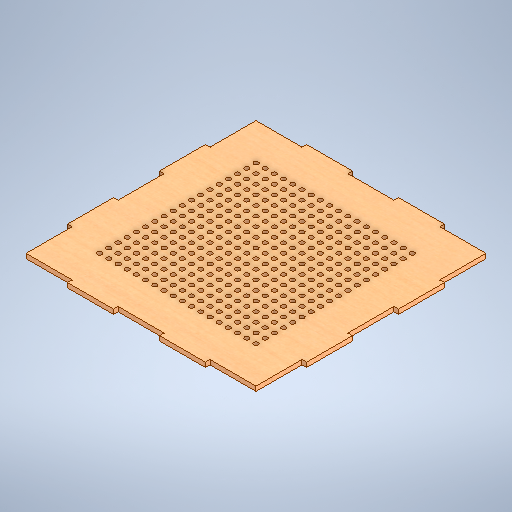
# Autodesk Inventor part: Tapa1
Saved by Autodesk Inventor 2025 (Build 290162000, 162)
## iProperties
Created: 2024-11-02
Part Number: Tapa1
Material: Wood (Cherry)
Document SubType Name: Sheet Metal
Designer: g.marin
Density: 0.63 g/cm^3
Sheet Metal Rule: Default
Appearance: Cherry - Natural Low Gloss
Author: g.marin
Autodesk Inventor part; units mm, degrees
ref_plane "YZ Plane" through (0, 0, 0) normal (1, 0, 0) x (0, 1, 0)
ref_plane "XZ Plane" through (0, 0, 0) normal (0, 1, 0) x (-1, 0, 0)
ref_plane "XY Plane" through (0, 0, 0) normal (0, 0, 1) x (1, 0, 0)
sketch "Sketch1" plane through (0, 0, 0) normal (0, 1, 0) x (-1, 0, 0)
  line L0 (-125, 125) -> (125, 125)
  line L1 (125, 125) -> (125, -125)
  line L2 (125, -125) -> (-125, -125)
  line L3 (-125, -125) -> (-125, 125)
  line L4 (-125, 125) -> (125, -125) construction
  line L5 (125, 125) -> (-125, -125) construction
  line L6 (0, 125) -> (0, -125) construction
  line L7 (125, 0) -> (-125, 0) construction
  line L8 (125, 75) -> (130, 75)
  line L9 (130, 75) -> (130, 25)
  line L10 (130, 25) -> (125, 25)
  line L11 (125, 25) -> (125, 75)
  line L12 (75, 125) -> (25, 125)
  line L13 (25, 125) -> (25, 130)
  line L14 (25, 130) -> (75, 130)
  line L15 (75, 130) -> (75, 125)
  line L16 (125, -75) -> (130, -75)
  line L17 (130, -75) -> (130, -25)
  line L18 (130, -25) -> (125, -25)
  line L19 (-125, 75) -> (-130, 75)
  line L20 (-130, 75) -> (-130, 25)
  line L21 (-130, 25) -> (-125, 25)
  line L22 (-130, -75) -> (-130, -25)
  line L23 (-125, -75) -> (-130, -75)
  line L24 (-130, -25) -> (-125, -25)
  line L25 (-25, 125) -> (-25, 130)
  line L26 (-25, 130) -> (-75, 130)
  line L27 (-75, 130) -> (-75, 125)
  line L28 (25, -125) -> (25, -130)
  line L29 (25, -130) -> (75, -130)
  line L30 (75, -130) -> (75, -125)
  line L31 (-75, -130) -> (-75, -125)
  line L32 (-25, -130) -> (-75, -130)
  line L33 (-25, -125) -> (-25, -130)
  line L34 (95, 95) -> (-95, 95)
  line L35 (-95, 95) -> (-95, -95)
  line L36 (-95, -95) -> (95, -95)
  line L37 (95, -95) -> (95, 95)
  line L38 (95, 95) -> (-95, -95) construction
  line L39 (-95, 95) -> (95, -95) construction
  circle A0 centre (85, -85) radius 2.5
  circle A1 centre (75, -85) radius 2.5
  circle A2 centre (65, -85) radius 2.5
  circle A3 centre (55, -85) radius 2.5
  circle A4 centre (45, -85) radius 2.5
  circle A5 centre (35, -85) radius 2.5
  circle A6 centre (25, -85) radius 2.5
  circle A7 centre (15, -85) radius 2.5
  circle A8 centre (5, -85) radius 2.5
  circle A9 centre (-5, -85) radius 2.5
  circle A10 centre (-15, -85) radius 2.5
  circle A11 centre (-25, -85) radius 2.5
  circle A12 centre (-35, -85) radius 2.5
  circle A13 centre (-45, -85) radius 2.5
  circle A14 centre (-55, -85) radius 2.5
  circle A15 centre (-65, -85) radius 2.5
  circle A16 centre (-75, -85) radius 2.5
  circle A17 centre (-85, -85) radius 2.5
  circle A18 centre (85, -75) radius 2.5
  circle A19 centre (75, -75) radius 2.5
  circle A20 centre (65, -75) radius 2.5
  circle A21 centre (55, -75) radius 2.5
  circle A22 centre (45, -75) radius 2.5
  circle A23 centre (35, -75) radius 2.5
  circle A24 centre (25, -75) radius 2.5
  circle A25 centre (15, -75) radius 2.5
  circle A26 centre (5, -75) radius 2.5
  circle A27 centre (-5, -75) radius 2.5
  circle A28 centre (-15, -75) radius 2.5
  circle A29 centre (-25, -75) radius 2.5
  circle A30 centre (-35, -75) radius 2.5
  circle A31 centre (-45, -75) radius 2.5
  circle A32 centre (-55, -75) radius 2.5
  circle A33 centre (-65, -75) radius 2.5
  circle A34 centre (-75, -75) radius 2.5
  circle A35 centre (-85, -75) radius 2.5
  circle A36 centre (85, -65) radius 2.5
  circle A37 centre (75, -65) radius 2.5
  circle A38 centre (65, -65) radius 2.5
  circle A39 centre (55, -65) radius 2.5
  circle A40 centre (45, -65) radius 2.5
  circle A41 centre (35, -65) radius 2.5
  circle A42 centre (25, -65) radius 2.5
  circle A43 centre (15, -65) radius 2.5
  circle A44 centre (5, -65) radius 2.5
  circle A45 centre (-5, -65) radius 2.5
  circle A46 centre (-15, -65) radius 2.5
  circle A47 centre (-25, -65) radius 2.5
  circle A48 centre (-35, -65) radius 2.5
  circle A49 centre (-45, -65) radius 2.5
  circle A50 centre (-55, -65) radius 2.5
  circle A51 centre (-65, -65) radius 2.5
  circle A52 centre (-75, -65) radius 2.5
  circle A53 centre (-85, -65) radius 2.5
  circle A54 centre (85, -55) radius 2.5
  circle A55 centre (75, -55) radius 2.5
  circle A56 centre (65, -55) radius 2.5
  circle A57 centre (55, -55) radius 2.5
  circle A58 centre (45, -55) radius 2.5
  circle A59 centre (35, -55) radius 2.5
  circle A60 centre (25, -55) radius 2.5
  circle A61 centre (15, -55) radius 2.5
  circle A62 centre (5, -55) radius 2.5
  circle A63 centre (-5, -55) radius 2.5
  circle A64 centre (-15, -55) radius 2.5
  circle A65 centre (-25, -55) radius 2.5
  circle A66 centre (-35, -55) radius 2.5
  circle A67 centre (-45, -55) radius 2.5
  circle A68 centre (-55, -55) radius 2.5
  circle A69 centre (-65, -55) radius 2.5
  circle A70 centre (-75, -55) radius 2.5
  circle A71 centre (-85, -55) radius 2.5
  circle A72 centre (85, -45) radius 2.5
  circle A73 centre (75, -45) radius 2.5
  circle A74 centre (65, -45) radius 2.5
  circle A75 centre (55, -45) radius 2.5
  circle A76 centre (45, -45) radius 2.5
  circle A77 centre (35, -45) radius 2.5
  circle A78 centre (25, -45) radius 2.5
  circle A79 centre (15, -45) radius 2.5
  circle A80 centre (5, -45) radius 2.5
  circle A81 centre (-5, -45) radius 2.5
  circle A82 centre (-15, -45) radius 2.5
  circle A83 centre (-25, -45) radius 2.5
  circle A84 centre (-35, -45) radius 2.5
  circle A85 centre (-45, -45) radius 2.5
  circle A86 centre (-55, -45) radius 2.5
  circle A87 centre (-65, -45) radius 2.5
  circle A88 centre (-75, -45) radius 2.5
  circle A89 centre (-85, -45) radius 2.5
  circle A90 centre (85, -35) radius 2.5
  circle A91 centre (75, -35) radius 2.5
  circle A92 centre (65, -35) radius 2.5
  circle A93 centre (55, -35) radius 2.5
  circle A94 centre (45, -35) radius 2.5
  circle A95 centre (35, -35) radius 2.5
  circle A96 centre (25, -35) radius 2.5
  circle A97 centre (15, -35) radius 2.5
  circle A98 centre (5, -35) radius 2.5
  circle A99 centre (-5, -35) radius 2.5
  circle A100 centre (-15, -35) radius 2.5
  circle A101 centre (-25, -35) radius 2.5
  circle A102 centre (-35, -35) radius 2.5
  circle A103 centre (-45, -35) radius 2.5
  circle A104 centre (-55, -35) radius 2.5
  circle A105 centre (-65, -35) radius 2.5
  circle A106 centre (-75, -35) radius 2.5
  circle A107 centre (-85, -35) radius 2.5
  circle A108 centre (85, -25) radius 2.5
  circle A109 centre (75, -25) radius 2.5
  circle A110 centre (65, -25) radius 2.5
  circle A111 centre (55, -25) radius 2.5
  circle A112 centre (45, -25) radius 2.5
  circle A113 centre (35, -25) radius 2.5
  circle A114 centre (25, -25) radius 2.5
  circle A115 centre (15, -25) radius 2.5
  circle A116 centre (5, -25) radius 2.5
  circle A117 centre (-5, -25) radius 2.5
  circle A118 centre (-15, -25) radius 2.5
  circle A119 centre (-25, -25) radius 2.5
  circle A120 centre (-35, -25) radius 2.5
  circle A121 centre (-45, -25) radius 2.5
  circle A122 centre (-55, -25) radius 2.5
  circle A123 centre (-65, -25) radius 2.5
  circle A124 centre (-75, -25) radius 2.5
  circle A125 centre (-85, -25) radius 2.5
  circle A126 centre (85, -15) radius 2.5
  circle A127 centre (75, -15) radius 2.5
  circle A128 centre (65, -15) radius 2.5
  circle A129 centre (55, -15) radius 2.5
  circle A130 centre (45, -15) radius 2.5
  circle A131 centre (35, -15) radius 2.5
  circle A132 centre (25, -15) radius 2.5
  circle A133 centre (15, -15) radius 2.5
  circle A134 centre (5, -15) radius 2.5
  circle A135 centre (-5, -15) radius 2.5
  circle A136 centre (-15, -15) radius 2.5
  circle A137 centre (-25, -15) radius 2.5
  circle A138 centre (-35, -15) radius 2.5
  circle A139 centre (-45, -15) radius 2.5
  circle A140 centre (-55, -15) radius 2.5
  circle A141 centre (-65, -15) radius 2.5
  circle A142 centre (-75, -15) radius 2.5
  circle A143 centre (-85, -15) radius 2.5
  circle A144 centre (85, -5) radius 2.5
  circle A145 centre (75, -5) radius 2.5
  circle A146 centre (65, -5) radius 2.5
  circle A147 centre (55, -5) radius 2.5
  circle A148 centre (45, -5) radius 2.5
  circle A149 centre (35, -5) radius 2.5
  circle A150 centre (25, -5) radius 2.5
  circle A151 centre (15, -5) radius 2.5
  circle A152 centre (5, -5) radius 2.5
  circle A153 centre (-5, -5) radius 2.5
  circle A154 centre (-15, -5) radius 2.5
  circle A155 centre (-25, -5) radius 2.5
  circle A156 centre (-35, -5) radius 2.5
  circle A157 centre (-45, -5) radius 2.5
  circle A158 centre (-55, -5) radius 2.5
  circle A159 centre (-65, -5) radius 2.5
  circle A160 centre (-75, -5) radius 2.5
  circle A161 centre (-85, -5) radius 2.5
  circle A162 centre (85, 5) radius 2.5
  circle A163 centre (75, 5) radius 2.5
  circle A164 centre (65, 5) radius 2.5
  circle A165 centre (55, 5) radius 2.5
  circle A166 centre (45, 5) radius 2.5
  circle A167 centre (35, 5) radius 2.5
  circle A168 centre (25, 5) radius 2.5
  circle A169 centre (15, 5) radius 2.5
  circle A170 centre (5, 5) radius 2.5
  circle A171 centre (-5, 5) radius 2.5
  circle A172 centre (-15, 5) radius 2.5
  circle A173 centre (-25, 5) radius 2.5
  circle A174 centre (-35, 5) radius 2.5
  circle A175 centre (-45, 5) radius 2.5
  circle A176 centre (-55, 5) radius 2.5
  circle A177 centre (-65, 5) radius 2.5
  circle A178 centre (-75, 5) radius 2.5
  circle A179 centre (-85, 5) radius 2.5
  circle A180 centre (85, 15) radius 2.5
  circle A181 centre (75, 15) radius 2.5
  circle A182 centre (65, 15) radius 2.5
  circle A183 centre (55, 15) radius 2.5
  circle A184 centre (45, 15) radius 2.5
  circle A185 centre (35, 15) radius 2.5
  circle A186 centre (25, 15) radius 2.5
  circle A187 centre (15, 15) radius 2.5
  circle A188 centre (5, 15) radius 2.5
  circle A189 centre (-5, 15) radius 2.5
  circle A190 centre (-15, 15) radius 2.5
  circle A191 centre (-25, 15) radius 2.5
  circle A192 centre (-35, 15) radius 2.5
  circle A193 centre (-45, 15) radius 2.5
  circle A194 centre (-55, 15) radius 2.5
  circle A195 centre (-65, 15) radius 2.5
  circle A196 centre (-75, 15) radius 2.5
  circle A197 centre (-85, 15) radius 2.5
  circle A198 centre (85, 25) radius 2.5
  circle A199 centre (75, 25) radius 2.5
  circle A200 centre (65, 25) radius 2.5
  circle A201 centre (55, 25) radius 2.5
  circle A202 centre (45, 25) radius 2.5
  circle A203 centre (35, 25) radius 2.5
  circle A204 centre (25, 25) radius 2.5
  circle A205 centre (15, 25) radius 2.5
  circle A206 centre (5, 25) radius 2.5
  circle A207 centre (-5, 25) radius 2.5
  circle A208 centre (-15, 25) radius 2.5
  circle A209 centre (-25, 25) radius 2.5
  circle A210 centre (-35, 25) radius 2.5
  circle A211 centre (-45, 25) radius 2.5
  circle A212 centre (-55, 25) radius 2.5
  circle A213 centre (-65, 25) radius 2.5
  circle A214 centre (-75, 25) radius 2.5
  circle A215 centre (-85, 25) radius 2.5
  circle A216 centre (85, 35) radius 2.5
  circle A217 centre (75, 35) radius 2.5
  circle A218 centre (65, 35) radius 2.5
  circle A219 centre (55, 35) radius 2.5
  circle A220 centre (45, 35) radius 2.5
  circle A221 centre (35, 35) radius 2.5
  circle A222 centre (25, 35) radius 2.5
  circle A223 centre (15, 35) radius 2.5
  circle A224 centre (5, 35) radius 2.5
  circle A225 centre (-5, 35) radius 2.5
  circle A226 centre (-15, 35) radius 2.5
  circle A227 centre (-25, 35) radius 2.5
  circle A228 centre (-35, 35) radius 2.5
  circle A229 centre (-45, 35) radius 2.5
  circle A230 centre (-55, 35) radius 2.5
  circle A231 centre (-65, 35) radius 2.5
  circle A232 centre (-75, 35) radius 2.5
  circle A233 centre (-85, 35) radius 2.5
  circle A234 centre (85, 45) radius 2.5
  circle A235 centre (75, 45) radius 2.5
  circle A236 centre (65, 45) radius 2.5
  circle A237 centre (55, 45) radius 2.5
  circle A238 centre (45, 45) radius 2.5
  circle A239 centre (35, 45) radius 2.5
  circle A240 centre (25, 45) radius 2.5
  circle A241 centre (15, 45) radius 2.5
  circle A242 centre (5, 45) radius 2.5
  circle A243 centre (-5, 45) radius 2.5
  circle A244 centre (-15, 45) radius 2.5
  circle A245 centre (-25, 45) radius 2.5
  circle A246 centre (-35, 45) radius 2.5
  circle A247 centre (-45, 45) radius 2.5
  circle A248 centre (-55, 45) radius 2.5
  circle A249 centre (-65, 45) radius 2.5
  circle A250 centre (-75, 45) radius 2.5
  circle A251 centre (-85, 45) radius 2.5
  circle A252 centre (85, 55) radius 2.5
  circle A253 centre (75, 55) radius 2.5
  circle A254 centre (65, 55) radius 2.5
  circle A255 centre (55, 55) radius 2.5
  circle A256 centre (45, 55) radius 2.5
  circle A257 centre (35, 55) radius 2.5
  circle A258 centre (25, 55) radius 2.5
  circle A259 centre (15, 55) radius 2.5
  circle A260 centre (5, 55) radius 2.5
  circle A261 centre (-5, 55) radius 2.5
  circle A262 centre (-15, 55) radius 2.5
  circle A263 centre (-25, 55) radius 2.5
  circle A264 centre (-35, 55) radius 2.5
  circle A265 centre (-45, 55) radius 2.5
  circle A266 centre (-55, 55) radius 2.5
  circle A267 centre (-65, 55) radius 2.5
  circle A268 centre (-75, 55) radius 2.5
  circle A269 centre (-85, 55) radius 2.5
  circle A270 centre (85, 65) radius 2.5
  circle A271 centre (75, 65) radius 2.5
  circle A272 centre (65, 65) radius 2.5
  circle A273 centre (55, 65) radius 2.5
  circle A274 centre (45, 65) radius 2.5
  circle A275 centre (35, 65) radius 2.5
  circle A276 centre (25, 65) radius 2.5
  circle A277 centre (15, 65) radius 2.5
  circle A278 centre (5, 65) radius 2.5
  circle A279 centre (-5, 65) radius 2.5
  circle A280 centre (-15, 65) radius 2.5
  circle A281 centre (-25, 65) radius 2.5
  circle A282 centre (-35, 65) radius 2.5
  circle A283 centre (-45, 65) radius 2.5
  circle A284 centre (-55, 65) radius 2.5
  circle A285 centre (-65, 65) radius 2.5
  circle A286 centre (-75, 65) radius 2.5
  circle A287 centre (-85, 65) radius 2.5
  circle A288 centre (85, 75) radius 2.5
  circle A289 centre (75, 75) radius 2.5
  circle A290 centre (65, 75) radius 2.5
  circle A291 centre (55, 75) radius 2.5
  circle A292 centre (45, 75) radius 2.5
  circle A293 centre (35, 75) radius 2.5
  circle A294 centre (25, 75) radius 2.5
  circle A295 centre (15, 75) radius 2.5
  circle A296 centre (5, 75) radius 2.5
  circle A297 centre (-5, 75) radius 2.5
  circle A298 centre (-15, 75) radius 2.5
  circle A299 centre (-25, 75) radius 2.5
  circle A300 centre (-35, 75) radius 2.5
  circle A301 centre (-45, 75) radius 2.5
  circle A302 centre (-55, 75) radius 2.5
  circle A303 centre (-65, 75) radius 2.5
  circle A304 centre (-75, 75) radius 2.5
  circle A305 centre (-85, 75) radius 2.5
  circle A306 centre (85, 85) radius 2.5
  circle A307 centre (75, 85) radius 2.5
  circle A308 centre (65, 85) radius 2.5
  circle A309 centre (55, 85) radius 2.5
  circle A310 centre (45, 85) radius 2.5
  circle A311 centre (35, 85) radius 2.5
  circle A312 centre (25, 85) radius 2.5
  circle A313 centre (15, 85) radius 2.5
  circle A314 centre (5, 85) radius 2.5
  circle A315 centre (-5, 85) radius 2.5
  circle A316 centre (-15, 85) radius 2.5
  circle A317 centre (-25, 85) radius 2.5
  circle A318 centre (-35, 85) radius 2.5
  circle A319 centre (-45, 85) radius 2.5
  circle A320 centre (-55, 85) radius 2.5
  circle A321 centre (-65, 85) radius 2.5
  circle A322 centre (-75, 85) radius 2.5
  circle A323 centre (-85, 85) radius 2.5
  point P0 (0, 0)
  point P1 (-25, 125)
  point P2 (-75, 125)
  point P3 (-125, -25)
  point P4 (-125, -75)
  point P5 (-75, -125)
  point P6 (-25, -125)
  point P7 (25, -125)
  point P8 (75, -125)
  point P9 (125, -75)
  point P10 (125, -25)
  point P11 (125, 25)
  dimension "d0" = 250
  dimension "d1" = 250
  dimension "d3" = 50
  dimension "d5" = 50
  dimension "d6" = 50
  dimension "d7" = 50
  dimension "d10" = 5
  dimension "d11" = 5
  dimension "d13" = 30
  dimension "d14" = 5
  dimension "d15" = 10
  dimension "d18" = 10
  dimension "d21" = 10
  constraints: 324 centre point, 80 end point, 24 symmetric about line, 8 midpoint, 8 parallel, 5 horizontal, 4 perpendicular, 4 point on line, 1 vertical, 646 other
  measures "d0" distance of L1.end L2.end
  measures "d1" distance of L0.end L1.end
  measures "d3" distance of L8.end L9.end
  measures "d5" distance between parallel lines of L15 L1
  measures "d6" distance between parallel lines of L0 L8
  measures "d7" distance of L13.end L14.end
  measures "d10" distance of L9.end L10.end
  measures "d11" distance of L12.end L13.end
  measures "d13" distance between parallel lines of L3 L35
  measures "d14" diameter of A0
  measures "d15" distance from line of A0.centre L36
  measures "d18" distance of A0.centre A1.centre
  measures "d21" distance of A0.centre A18.centre
extrude "Extrusion1" add sketch "Sketch1" along normal blind 5 contours L0 L1 L2 L3 | L27 L26 L25 L0 | L3 L21 L20 L19 | L13 L14 L15 L0 | L3 L23 L22 L24 | L8 L9 L10 L1 | L2 L33 L32 L31 | L18 L17 L16 L1 | L2 L30 L29 L28 | L37 L36 L35 L34
equation "\"BendRadius\" = Thickness"
equation "\"BendReliefWidth\" = Thickness"
equation "\"BendReliefDepth\" = 0.5 * Thickness"
equation "\"CornerReliefSize\" = 4 * Thickness"
equation "\"MinimumRemnant\" = 2 * Thickness"
equation "\"TransitionRadius\" = BendRadius"
equation "\"JacobiRadiusSize\" = BendRadius"
equation "\"GapSize\" = Thickness"
equation "\"Thickness\" = 3.048"
body "Solid1"
